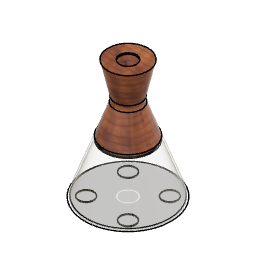
forme-maj-2023-12-19-c-ache-impression-3d v2 (Autodesk Fusion 360 design; units mm, degrees)
Autodesk Fusion 360 part; units mm, degrees
sketch "Esquisse1" plane through (0, 0, 0) normal (0, 0, 1) x (1, 0, 0)
  line L0 (0, 0) -> (-65, 0)
  line L1 (-65, 0) -> (-36, 80)
  line L2 (-36, 80) -> (0, 80)
  line L3 (0, 80) -> (0, 0)
  dimension "d1" = 65
  dimension "d2" = 36
  dimension "d3" = 80
  constraint coincident L0.start L3.end
  constraint horizontal L0
  constraint parallel L0 L2
  constraint perpendicular L0 L3
  measures "d1" distance of L0.start L0.end
  measures "d2" distance of L1.end L2.end
  measures "d3" vertical distance of L0.end L1.end
revolve "Révolution1" add sketch "Esquisse1" angle 360 about axis through (0, 80, 0) along (0, -1, 0) makes body 1
shell "Coque1" thickness 2 removed faces 1 at (-7.6159, 80, -11.1705) on bodies 1
sketch "Esquisse2" plane through (0, 0, 0) normal (0, 0, 1) x (1, 0, 0)
  line L0 (0, 80) -> (-36, 80)
  line L1 (-36, 80) -> (-20.0913, 123.8862)
  line L2 (-19.5546, 132.2704) -> (-30, 179)
  line L3 (-30, 179) -> (0, 179)
  line L4 (0, 179) -> (0, 80)
  arc A0 (-20.0913, 123.8862) -> (-19.5546, 132.2704) centre (-34.1933, 128.9982) ccw
  line L5 (0, 1.75) -> (0, 22.5)
  line L6 (-19.5546, 132.2704) -> (-18.6, 128) construction
  line L7 (-18.6, 128) -> (-20.0913, 123.8862) construction
  line L8 (65, 0) -> (-65, 0)
  line L9 (36, 80) -> (-36, 80)
  line L10 (-65, 0) -> (-36, 80)
  line L11 (-36, 80) -> (0, 80)
  point P0 (-18.6, 128)
  point P1 (-36, 80)
  dimension "d6" = 30
  dimension "d8" = 48
  dimension "d9" = 51
  dimension "d10" = 15
  dimension "d44" = 18.6
  dimension "d45" = 36
  constraint horizontal L0
  constraint horizontal L3
  constraint perpendicular L0 L4
  constraint coincident P0 L1
  constraint coincident P0 L2
  constraint tangent L1 A0
  constraint tangent L2 A0
  constraint collinear L4 L5
  constraint coincident P0 L6.end
  constraint parallel L1 L10
  constraint coincident P1 L0.end
  measures "d6" distance of L2.end L3.end
  measures "d8" vertical distance of P1 P0
  measures "d9" vertical distance of P0 L2.end
  measures "d10" radius of A0
  measures "d44" distance of P0 L4
  measures "d45" distance of P1 L0.start
revolve "Révolution2" add sketch "Esquisse2" angle 360 about axis through (0, 179, 0) along (0, -1, 0) separate body makes body 2
sketch "Esquisse6" plane through (0, 0, 0) normal (0, 0, 1) x (1, 0, 0)
  line L0 (-33.8726, 80) -> (-35.6851, 80)
  line L1 (-35.6851, 80) -> (-35.6851, 75)
  line L2 (-35.6851, 75) -> (-33.8726, 75)
  line L3 (-33.8726, 75) -> (-33.8726, 80)
  line L4 (62.1476, 2) -> (-62.1476, 2)
  line L5 (-33.8726, 80) -> (33.8726, 80)
  line L6 (-62.1476, 2) -> (-33.8726, 80) construction
  dimension "d46" = 5
  constraint horizontal L0
  constraint vertical L1
  constraint horizontal L2
  constraint vertical L3
  constraint coincident L4.end L6.start
  constraint coincident L0.start L3.end
  constraint coincident L1.end L6
  measures "d46" distance of L0.start L2.end
revolve "Révolution4" add sketch "Esquisse6" angle 360 about axis through (0, 1.75, 0) along (0, 1, 0) bodies 1
sketch "Esquisse3" plane through (0, 0, 0) normal (0, 0, 1) x (1, 0, 0)
  line L0 (-33.7226, 80) -> (-33.7226, 75)
  line L1 (-33.7226, 75) -> (-31.2226, 75)
  line L2 (-31.2226, 75) -> (-31.2226, 80)
  line L3 (-31.2226, 80) -> (-33.7226, 80)
  line L4 (30, 179) -> (-30, 179)
  line L5 (36, 80) -> (-36, 80)
  arc A0 (-20.0913, 123.8862) -> (-19.5546, 132.2704) centre (-34.1933, 128.9982) ccw
  arc A1 (19.5546, 132.2704) -> (20.0913, 123.8862) centre (34.1933, 128.9982) ccw
  line L6 (19.5546, 132.2704) -> (30, 179)
  line L7 (-19.5546, 132.2704) -> (-30, 179)
  line L8 (-20.0913, 123.8862) -> (-36, 80)
  line L9 (20.0913, 123.8862) -> (36, 80)
  point P0 (-33.8726, 80)
  dimension "d12" = 5
  dimension "d13" = 2.5
  dimension "d48" = 0.15
  constraint vertical L0
  constraint perpendicular L0 L1
  constraint perpendicular L1 L2
  constraint perpendicular L0 L3
  constraint collinear L3 L5
  measures "d12" distance of L0.start L0.end
  measures "d13" distance of L0.end L1.end
  measures "d48" distance of L0 P0
revolve "Révolution3" add sketch "Esquisse3" angle 360 about axis through (0, 1.75, 0) along (0, 1, 0) contours L0 L1 L2 L3 L5 bodies 2
shell "Coque3" thickness 2 removed faces 1 at (5.0026, 80, -11.6978) on bodies 2
hole "Perçage1" at (0, 179, 0) direction (0, -1, 0) diameter 25.3 depth 100 tip angle 180 bodies 2
sketch "Esquisse7" plane through (0, 0, 0) normal (0, -1, 0) x (1, 0, 0)
  circle A0 centre (0, 0) radius 65
  circle A1 centre (-31.6322, 31.6322) radius 11.25
  circle A2 centre (-31.6322, -31.6322) radius 11.25
  circle A3 centre (31.6322, 31.6322) radius 11.25
  circle A4 centre (31.6322, -31.6322) radius 11.25
  line L0 (-31.6322, 31.6322) -> (31.6322, -31.6322) construction
  line L1 (-31.6322, -31.6322) -> (31.6322, 31.6322) construction
  line L2 (-31.6322, 31.6322) -> (31.6322, 31.6322) construction
  line L3 (31.6322, 31.6322) -> (31.6322, -31.6322) construction
  line L4 (31.6322, -31.6322) -> (-31.6322, -31.6322) construction
  line L5 (-31.6322, -31.6322) -> (-31.6322, 31.6322) construction
  dimension "d49" = 22.5
  constraint horizontal A1.centre A3.centre
  constraint horizontal A2.centre A4.centre
  constraint vertical A1.centre A2.centre
  constraint vertical A3.centre A4.centre
  constraint coincident A1.centre L0.start
  constraint coincident A4.centre L0.end
  constraint coincident A2.centre L1.start
  constraint coincident A3.centre L1.end
  constraint midpoint A0.centre L0
  constraint horizontal L2
  constraint vertical L3
  constraint horizontal L4
  constraint vertical L5
  constraint equal L2 L3
  constraint equal A1 A3
  constraint equal A1 A4
  constraint equal A1 A2
  measures "d49" diameter of A3
extrude "Extrusion3" cut sketch "Esquisse7" against normal blind 1 contours A1 | A2 | A3 | A4 bodies 1
extrude "Extrusion4" add 1 faces at (31.3216, 80, -3.1272) along direction (0, 1, 0) up to surface (2 mm away) on bodies 2 bodies 2
equation "d2 = 38 mm - 2 mm"
equation "d17 = 25 mm + 0.30 mm"
equation "d48 = ( 0.3 / 2 ) * 1 mm"
named bodies: "Partie basse Pion résine", "Partie haute Pion bois"
